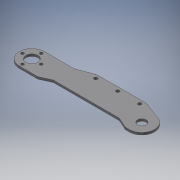
# Autodesk Inventor part: rinnku
Saved by Autodesk Inventor 2018 (Build 220112000, 112)
## iProperties
Created: 2016-08-23
Part Number: rinnku
Material: GFRP
Document SubType Name: Modeling
Designer: hiro
Density: 1.75 g/cm^3
Appearance: 滑らか - 淡い灰色
Mass: 9.22094 g
Surface Area: 59.6576 cm^2
Volume: 5.26911 cm^3
Author: hiro
Autodesk Inventor part; units mm, degrees
ref_plane "YZ Plane" through (0, 0, 0) normal (1, 0, 0) x (0, 1, 0)
ref_plane "XZ Plane" through (0, 0, 0) normal (0, 1, 0) x (-1, 0, 0)
ref_plane "XY Plane" through (0, 0, 0) normal (0, 0, 1) x (1, 0, 0)
sketch "スケッチ1" plane through (0, 0, 0) normal (0, 0, 1) x (1, 0, 0)
  line L0 (-50, 0) -> (50, 0) construction
  circle A0 centre (-50, 0) radius 5.5
  circle A1 centre (50, 0) radius 4
  line L1 (-50, 11.35) -> (50, 11.35)
  line L2 (-50, -11.35) -> (50, -11.35)
  arc A2 (-50, 11.35) -> (-50, -11.35) centre (-50, 0) ccw
  arc A3 (50, -11.35) -> (50, 11.35) centre (50, 0) ccw
  line L3 (53.987, 10.6267) -> (37, 17)
  line L4 (37, 17) -> (-8, 17)
  line L5 (-11.9652, 10) -> (55.6573, 10) construction
  line L6 (-8, 17) -> (-8, 10) construction
  line L7 (37, 17) -> (37, 10) construction
  circle A4 centre (34.5, 13.5) radius 1.55
  circle A5 centre (-5.5, 13.5) radius 1.55
  circle A6 centre (14.5, 13.5) radius 1.55
  line L8 (-8, 13.5) -> (37, 13.5) construction
  line L9 (37, 16) -> (-8, 16) construction
  line L10 (-8, 16) -> (-8, 11) construction
  line L11 (-8, 11) -> (37, 11) construction
  line L12 (37, 11) -> (37, 16) construction
  line L13 (-8, 17) -> (-23.0591, 11.35)
  line L14 (14.5, 17) -> (14.5, 3.4639) construction
  point P0 (0, 0)
  point P1 (0, 0)
  point P2 (-11.3055, 11.35)
  dimension "d0" = 100
  dimension "d1" = 11
  dimension "d2" = 11.35
  dimension "d8" = 8
  dimension "d10" = 7
  dimension "d11" = 45
  dimension "d12" = 2.5
  dimension "d13" = 3.1
  dimension "d14" = 2.5
  dimension "d15" = 13
  dimension "d17" = 5
  dimension "d18" = 11
  constraints: 30 end point, 9 point on line, 7 centre point, 6 horizontal, 6 midpoint, 5 coincident, 5 point on circle, 4 perpendicular, 4 tangent, 2 equal radius, 2 parallel, 1 other
  measures "d0" distance of L0.start L0.end
  measures "d1" diameter of A0
  measures "d2" radius of A2
  measures "d8" diameter of A1
  measures "d10" distance between parallel lines of L4 L5
  measures "d11" distance between parallel lines of L7 L6
  measures "d12" distance from line of A5.centre L6
  measures "d13" diameter of A5
  measures "d14" distance from line of L7 A4.centre
  measures "d15" distance from line of L7 L0.end
  measures "d17" distance between parallel lines of L9 L11
  measures "d18" distance between parallel lines of L0 L11
extrude "押し出し1" add sketch "スケッチ1" along normal blind 2
fillet "フィレット1" radius 5 3 edges at (-8, 17, 1) (37, 17, 1) (-23.0591, 11.35, 1)
sketch "スケッチ2" plane through (0, 0, 2) normal (0, 0, 1) x (1, 0, 0)
  arc A0 (50, -11.35) -> (53.987, 10.6267) centre (50, 0) ccw projected
  line L0 (18, -20) -> (-35.4549, -20) construction
  line L1 (-76.9372, -11.5) -> (-72, -11.5)
  line L2 (-76.9372, -12.4) -> (-76.9372, -11.5)
  line L3 (-71.9872, -11.45) -> (-76.9872, -11.45)
  line L4 (-76.9872, -11.45) -> (-76.9872, -12.45)
  circle A1 centre (-50, 0) radius 5.5 projected
  circle A2 centre (-50, 0) radius 5.5 construction
  circle A3 centre (50, 0) radius 4 projected
  line L5 (83.3205, -17.7128) -> (50, 0) construction
  line L6 (50, 0) -> (18, -20) construction
  line L7 (83.3205, -17.7128) -> (37.8533, -17.7128) construction
  line L8 (-23.4166, -12.4128) -> (36.4577, -12.4128)
  line L9 (36.4577, -12.4128) -> (36.4577, -11.5128)
  line L10 (36.4577, -11.5128) -> (46.5205, -11.5128)
  line L11 (46.5205, -11.5128) -> (36.5205, -7.0128)
  line L12 (36.5205, -7.0128) -> (-23.4795, -7.0128)
  line L13 (-23.4795, -7.0128) -> (-33.4795, -11.5128)
  line L14 (-33.4795, -11.5128) -> (-23.4166, -11.5128)
  line L15 (-23.4166, -11.5128) -> (-23.4166, -12.4128)
  line L16 (-33.4902, -11.4628) -> (-23.4902, -6.9628)
  line L17 (-23.4902, -6.9628) -> (36.5312, -6.9628)
  line L18 (36.5312, -6.9628) -> (46.5312, -11.4628)
  line L19 (46.5312, -11.4628) -> (36.5077, -11.4628)
  line L20 (36.5077, -11.4628) -> (36.5077, -12.4628)
  line L21 (36.5077, -12.4628) -> (-23.4666, -12.4628)
  line L22 (-23.4666, -12.4628) -> (-23.4666, -11.4628)
  line L23 (-23.4666, -11.4628) -> (-33.4902, -11.4628)
  point P0 (0, 0)
  dimension "d19" = 20
  dimension "d20" = 32
  dimension "d32" = 11
  dimension "d33" = 120
  dimension "d37" = 36.8
  dimension "d38" = 6.2
  dimension "d39" = 0.05
  dimension "d49" = 60
  dimension "d50" = 10
  dimension "d51" = 10
  dimension "d52" = 4.5
  dimension "d53" = 0.9
  dimension "d54" = 59.9743
  constraints: 48 end point, 6 horizontal, 4 perpendicular, 3 equal length, 2 collinear, 1 centre point, 1 coincident, 1 horizontal alignment, 8 other
  measures "d19" vertical distance of A0.centre L0.start
  measures "d20" horizontal distance of L0.start A0.centre
  measures "d32" diameter of A2
  measures "d33" angle of L6 L5
  measures "d37" horizontal distance of L5.start L10.end
  measures "d38" distance from line of L10 L5.start
  measures "d39" distance between parallel lines of L16 L13
  measures "d49" distance of L11.end L12.end
  measures "d50" horizontal distance of L12.end L13.end
  measures "d51" horizontal distance of L10.end L11.end
  measures "d52" distance from line of L10.end L12
  measures "d53" distance between parallel lines of L8 L10
  measures "d54" distance between parallel lines of L22 L20
extrude "押し出し2" cut sketch "スケッチ2" against normal blind 10 contours L15 L14 L22 L23 L13 L12 L11 L19 L20 L10 L9 L8 | L8 L9 L10 L20 L21 L22 L14 L15 | L23 L16 L17 L18 L19 L11 L12 L13
fillet "フィレット2" radius 2 4 edges at (-33.2395, -11.35, 1) (-23.4902, -6.9628, 1) (46.2805, -11.35, 1) (36.5312, -6.9628, 1)
sketch "スケッチ3" plane through (0, 0, 2) normal (0, 0, 1) x (1, 0, 0)
  arc A0 (-50, 11.35) -> (-50, -11.35) centre (-50, 0) ccw projected
  circle A1 centre (-50, 0) radius 5.5 projected
  circle A2 centre (-50, 0) radius 8.5 construction
  circle A3 centre (-50, 8.5) radius 1.35
  line L0 (-50, 0) -> (-50, 8.5) construction
  line L1 (-50, 0) -> (-58.5, 0) construction
  circle A4 centre (-58.5, 0) radius 1.35
  line L2 (-50, 0) -> (-50, -8.5) construction
  circle A5 centre (-50, -8.5) radius 1.35
  line L3 (-50, 0) -> (-41.5, 0) construction
  circle A6 centre (-41.5, 0) radius 1.35
  point P0 (0, 0)
  dimension "d40" = 17
  dimension "d41" = 2.7
  dimension "d44" = 360
  constraints: 8 end point, 4 centre point, 1 coincident, 1 vertical, 1 vertical alignment, 19 other
  measures "d41" diameter of A3
extrude "押し出し3" cut sketch "スケッチ3" against normal blind 10 contours A3 | A4 | A5 | A6
equation "\"d14\" = d12"
